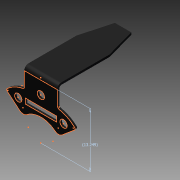
# Autodesk Inventor part: ASAP_Top_Fixture_Handle_New
Saved by Autodesk Inventor 2011 SP2 (Build 150309200, 309)
## iProperties
Created: 2011-11-18
Part Number: ASAP_Top_Fixture_Handle_New
Material: Default
Document SubType Name: Sheet Metal
Designer: sungwook
Density: 1 g/cm^3
Sheet Metal Rule: Default_mm
Flat Pattern Width: 1.65997 cm
Flat Pattern Length: 2.93845 cm
Flat Pattern Area: 4.87773 cm^2
Sheet Metal Width: 16.600 mm
Sheet Metal Length: 29.385 mm
Sheet Metal Area: 487.773 mm^2
Author: sungwook
Autodesk Inventor part; units mm, degrees
ref_plane "YZ Plane" through (0, 0, 0) normal (1, 0, 0) x (0, 1, 0)
ref_plane "XZ Plane" through (0, 0, 0) normal (0, 1, 0) x (-1, 0, 0)
ref_plane "XY Plane" through (0, 0, 0) normal (0, 0, 1) x (1, 0, 0)
sketch "Sketch1" plane through (0, 0, 0) normal (0, 0, 1) x (1, 0, 0)
  line L0 (-4, 10) -> (4, 10)
  line L1 (4, 10) -> (4, -10)
  line L2 (4, -10) -> (-4, -10)
  line L3 (-4, -10) -> (-4, 10)
  line L4 (-2, 10) -> (-4, 2.68)
  line L5 (0, -14) -> (0, 14)
  line L6 (2, 10) -> (4, 2.68)
  point P0 (0, 0)
  point P1 (0, 10)
  point P2 (-4, 0)
  dimension "d0" = 8
  dimension "d1" = 20
  dimension "d2" = 7.32
  dimension "d3" = 2
  dimension "d4" = 7.32
  dimension "d5" = 4
  measures "d0" distance between parallel lines of L1 L3
  measures "d1" distance between parallel lines of L2 L0
  measures "d2" vertical distance of L4.end L4.start
  measures "d3" distance of point (0, 10) L4.start
  measures "d4" vertical distance of L6.end L6.start
  measures "d5" distance of L6.start L4.start
extrude "Plate1" add sketch "Sketch1" along normal blind 0.508 contours L0 L5 L2 L3 L4 | L0 L6 L1 L2 L5
sketch "Sketch2" plane through (-4, -9.492, 0.508) normal (0, -1, 0) x (1, 0, 0)
  line L0 (8, 0) -> (0, 0)
  line L1 (0, 0) -> (0, -5)
  line L2 (0, -5) -> (8, -5)
  line L3 (8, -5) -> (8, 0)
  constraints: 4 end point, 4 other
edge flange "Flange1" height 5 angle 90 thickness 0.508 bend radius 0.508 thickness toward (0, -1, 0) relief straight relief width 0.508 relief depth 0.254 edges at (0, -10, 0) wall of the first edge with corners at (4, -9.492, 0.508) (-4, -9.492, 0.508) (-4, -9.492, -4.492) (4, -9.492, -4.492)
bend "Bend1"
corner "Corner1"
sketch "Block1" plane through (0, 0, 0) normal (0, 0, 1) x (1, 0, 0)
  line L0 (7.81, 3.3711) -> (7.81, 2.1011)
  circle A0 centre (12.3485, 0.5711) radius 0.5969
  arc A1 (12.9709, 2.3131) -> (7.0007, 5.198) centre (7.0007, -2.422) ccw
  arc A2 (14.6474, -0.5905) -> (12.9709, 2.3131) centre (4, -4.802) ccw
  circle A3 centre (10.0622, -0.7489) radius 0.8509
  line L1 (7.0007, 5.198) -> (0.9993, 5.198)
  arc A4 (14.1606, -7.2033) -> (14.6474, -0.5905) centre (7.5615, -3.3933) ccw
  line L2 (0.19, 2.1011) -> (0.19, 3.3711)
  line L3 (0.19, 3.3711) -> (7.81, 3.3711)
  line L4 (7.81, 2.1011) -> (0.19, 2.1011)
  arc A5 (7.9034, -8.1237) -> (9.3073, -5.692) centre (9.0593, -7.1699) ccw
  line L5 (11.1599, -12.4007) -> (14.1606, -7.2033)
  arc A6 (9.3073, -5.692) -> (7.9034, -8.1237) centre (4, -4.2489) ccw
  arc A7 (5.6764, -16.1286) -> (11.1599, -12.4007) centre (4.5608, -8.5907) ccw
  circle A8 centre (4, -11.2489) radius 0.8509
  circle A9 centre (4, -13.8889) radius 0.5969
  arc A10 (2.3236, -16.1286) -> (5.6764, -16.1286) centre (4, -4.802) ccw
  line L6 (-6.1606, -7.2033) -> (-3.1599, -12.4007)
  arc A11 (-3.1599, -12.4007) -> (2.3236, -16.1286) centre (3.4392, -8.5907) ccw
  arc A12 (0.9993, 5.198) -> (-4.9709, 2.3131) centre (0.9993, -2.422) ccw
  circle A13 centre (-2.0622, -0.7489) radius 0.8509
  arc A14 (-6.6474, -0.5905) -> (-6.1606, -7.2033) centre (0.4385, -3.3933) ccw
  arc A15 (-4.9709, 2.3131) -> (-6.6474, -0.5905) centre (4, -4.802) ccw
  circle A16 centre (-4.3485, 0.5711) radius 0.5969
  line L7 (4, -4.802) -> (4, 5.198)
  point P0 (4.4036, -3.4113)
sketch "Sketch13" plane through (-4, -10, -4.492) normal (0, -1, 0) x (1, 0, 0)
  line L0 (8, 3.984) -> (0, 3.984) projected
  line L1 (4, -27.1268) -> (4, 10.3545) projected
  circle A0 centre (4, -9.2649) radius 11.5
  line L2 (7.81, -1.6449) -> (7.81, -2.9149)
  circle A1 centre (12.3485, -4.4449) radius 0.5969
  arc A2 (12.9709, -2.7029) -> (7.0007, 0.182) centre (7.0007, -7.438) ccw
  arc A3 (14.6474, -5.6065) -> (12.9709, -2.7029) centre (4, -9.818) ccw
  circle A4 centre (10.0622, -5.7649) radius 0.8509
  line L3 (7.0007, 0.182) -> (0.9993, 0.182)
  arc A5 (14.1606, -12.2193) -> (14.6474, -5.6065) centre (7.5615, -8.4093) ccw
  line L4 (0.19, -2.9149) -> (0.19, -1.6449)
  line L5 (0.19, -1.6449) -> (7.81, -1.6449)
  line L6 (7.81, -2.9149) -> (0.19, -2.9149)
  arc A6 (7.9034, -13.1397) -> (9.3073, -10.708) centre (9.0593, -12.1859) ccw
  line L7 (11.1599, -17.4167) -> (14.1606, -12.2193)
  arc A7 (9.3073, -10.708) -> (7.9034, -13.1397) centre (4, -9.2649) ccw
  arc A8 (5.6764, -21.1446) -> (11.1599, -17.4167) centre (4.5608, -13.6067) ccw
  circle A9 centre (4, -16.2649) radius 0.8509
  circle A10 centre (4, -18.9049) radius 0.5969
  arc A11 (2.3236, -21.1446) -> (5.6764, -21.1446) centre (4, -9.818) ccw
  line L8 (-6.1606, -12.2193) -> (-3.1599, -17.4167)
  arc A12 (-3.1599, -17.4167) -> (2.3236, -21.1446) centre (3.4392, -13.6067) ccw
  arc A13 (0.9993, 0.182) -> (-4.9709, -2.7029) centre (0.9993, -7.438) ccw
  circle A14 centre (-2.0622, -5.7649) radius 0.8509
  arc A15 (-6.6474, -5.6065) -> (-6.1606, -12.2193) centre (0.4385, -8.4093) ccw
  arc A16 (-4.9709, -2.7029) -> (-6.6474, -5.6065) centre (4, -9.818) ccw
  circle A17 centre (-4.3485, -4.4449) radius 0.5969
  line L9 (4, -9.818) -> (4, 0.182)
  point P0 (4, 4.492)
  point P1 (4, 3.984)
  dimension "d79" = 3.802
  dimension "d83" = 13.249
  dimension "d110" = 23
  constraints: 1 centre point, 1 midpoint, 1 point on line, 1 other
  measures "d110" diameter of A0
sketch "Sketch15" plane through (-4, -10, -4.492) normal (0, -1, 0) x (1, 0, 0)
  line L0 (0, 0) -> (0, 3.984)
  arc A0 (9.3073, -10.708) -> (7.9034, -13.1397) centre (4, -9.2649) ccw
  arc A1 (0.9993, 0.182) -> (-4.9709, -2.7029) centre (0.9993, -7.438) ccw
  circle A2 centre (-4.3485, -4.4449) radius 0.5969
  circle A3 centre (-2.0622, -5.7649) radius 0.8509
  line L1 (4, -21.0244) -> (4, 9.3374)
  arc A4 (-4.125, -1.8061) -> (-4.165, -2.4137) centre (-3.9224, -2.1246) ccw
  arc A5 (-0.4226, 0.0482) -> (0, 0.5585) centre (-0.5195, 0.5585) ccw
  arc A6 (-1.1371, -4.9544) -> (0.5601, -4.9734) centre (-0.2769, -3.9292) ccw
  arc A7 (-0.4226, 0.0482) -> (-4.125, -1.8061) centre (1.0102, -7.4359) ccw
  line L2 (0, 0.5585) -> (4, 0.5585)
  arc A8 (4, -3.7649) -> (0.5601, -4.9734) centre (4, -9.2649) ccw
  line L3 (-1.1371, -4.9544) -> (-4.165, -2.4137)
  arc A9 (12.165, -2.4137) -> (12.125, -1.8061) centre (11.9224, -2.1246) ccw
  arc A10 (8, 0.5585) -> (8.4226, 0.0482) centre (8.5195, 0.5585) ccw
  arc A11 (7.4399, -4.9734) -> (9.1371, -4.9544) centre (8.2769, -3.9292) ccw
  arc A12 (12.125, -1.8061) -> (8.4226, 0.0482) centre (6.9898, -7.4359) ccw
  line L4 (8, 0.5585) -> (4, 0.5585)
  arc A13 (7.4399, -4.9734) -> (4, -3.7649) centre (4, -9.2649) ccw
  line L5 (9.1371, -4.9544) -> (12.165, -2.4137)
  line L6 (4, -9.2649) -> (-6.1438, -0.7533)
  point P0 (4, 4.492)
  dimension "d112" = 50
  measures "d112" angle of L1 L6
sheet face with bend "Face5" sketch "Sketch15" thickness 0.508 toward (0, 1, 0) bend radius 0.508 relief straight relief width 0.508 relief depth 0.254 contours A1 A5 L0 | L0 L2 L1 A0 A6 L3 A4 A7 A1 | A7 A4 A1 | L4 A10 A12 A9 L5 A11 A0 L1
bend "Bend6"
extrude "Cut2" cut sketch "Sketch13" against normal blind 0.508 contours L5 L2 L6 L1 | L1 L6 L4 L5
sketch "Sketch16" plane through (-4, -10, -0.508) normal (0, -1, 0) x (1, 0, 0)
  line L0 (4, -16.1019) -> (4, 3.869) projected
  point P0 (0.19, -6.8989)
  point P1 (4, 0.508)
  point P2 (-1.5, -6.3989)
  dimension "d92" = 5.5
  dimension "d94" = 0.5
  measures "d92" distance from line of L0 point (-1.5, -6.399)
  measures "d94" vertical distance of point (-1.5, -6.399) point (0.19, -6.899)
hole "Hole3" at (-5.5, -10, -6.9069) direction (0, 1, 0) diameter 1.778 end through all clearance for "Flat Head Machine Screw (82)" size "#0" standard "Ansi Unified Screw Threads"
mirror "Mirror2" about plane through (0, 0, 0) normal (1, 0, 0) of "Hole3"
sketch "Sketch17" plane through (-4, -10, -0.508) normal (0, -1, 0) x (1, 0, 0)
  line L0 (0.19, -5.6289) -> (7.81, -5.6289) projected
  point P0 (4, 0.508)
  point P1 (4, -3.1289)
  dimension "d102" = 2.5
  measures "d102" distance from line of point (4, -3.129) L0
hole "Hole4" at (0, -10, -3.6369) direction (0, 1, 0) diameter 1.778 end through all clearance for "Flat Head Machine Screw (82)" size "#0" standard "Ansi Unified Screw Threads"
sketch "Sketch18" plane through (-4, -10, -0.508) normal (0, -1, 0) x (1, 0, 0)
  circle A0 centre (4, -3.1289) radius 0.889 projected
  circle A1 centre (9.5, -6.3989) radius 0.889 projected
  circle A2 centre (-1.5, -6.3989) radius 0.889 projected
  line L0 (7.81, -5.6289) -> (7.81, -6.8989) projected
  line L1 (7.81, -6.8989) -> (0.19, -6.8989) projected
  line L2 (0.19, -6.8989) -> (0.19, -5.6289) projected
  line L3 (0.19, -5.6289) -> (7.81, -5.6289) projected
  line L4 (8, 0) -> (8, -3.4255) projected
  line L5 (8, 0) -> (0, 0) projected
  line L6 (0, -3.4255) -> (0, 0) projected
  arc A3 (-0.4226, -3.9358) -> (0, -3.4255) centre (-0.5195, -3.4255) ccw projected
  arc A4 (-0.4226, -3.9358) -> (-4.125, -5.7901) centre (1.0102, -11.4199) ccw projected
  arc A5 (-4.125, -5.7901) -> (-4.165, -6.3977) centre (-3.9224, -6.1086) ccw projected
  line L7 (-4.165, -6.3977) -> (-1.1371, -8.9384) projected
  arc A6 (-1.1371, -8.9384) -> (0.5601, -8.9574) centre (-0.2769, -7.9132) ccw projected
  arc A7 (7.4399, -8.9574) -> (0.5601, -8.9574) centre (4, -13.2489) ccw projected
  arc A8 (7.4399, -8.9574) -> (9.1371, -8.9384) centre (8.2769, -7.9132) ccw projected
  line L8 (9.1371, -8.9384) -> (12.165, -6.3977) projected
  arc A9 (12.165, -6.3977) -> (12.125, -5.7901) centre (11.9224, -6.1086) ccw projected
  arc A10 (12.125, -5.7901) -> (8.4226, -3.9358) centre (6.9898, -11.4199) ccw projected
  arc A11 (8, -3.4255) -> (8.4226, -3.9358) centre (8.5195, -3.4255) ccw projected
  point P0 (4, 0.508)
sketch "Sketch19" plane through (-4, -10, -0.508) normal (0, -1, 0) x (1, 0, 0)
  circle A0 centre (4, -3.1289) radius 0.889 projected
  circle A1 centre (9.5, -6.3989) radius 0.889 projected
  circle A2 centre (-1.5, -6.3989) radius 0.889 projected
  line L0 (7.81, -5.6289) -> (7.81, -6.8989) projected
  line L1 (7.81, -6.8989) -> (0.19, -6.8989) projected
  line L2 (0.19, -6.8989) -> (0.19, -5.6289) projected
  line L3 (0.19, -5.6289) -> (7.81, -5.6289) projected
  line L4 (8, 0) -> (8, -3.4255) projected
  line L5 (8, 0) -> (0, 0) projected
  line L6 (0, -3.4255) -> (0, 0) projected
  arc A3 (-0.4226, -3.9358) -> (0, -3.4255) centre (-0.5195, -3.4255) ccw projected
  arc A4 (-0.4226, -3.9358) -> (-4.125, -5.7901) centre (1.0102, -11.4199) ccw projected
  arc A5 (-4.125, -5.7901) -> (-4.165, -6.3977) centre (-3.9224, -6.1086) ccw projected
  line L7 (-4.165, -6.3977) -> (-1.1371, -8.9384) projected
  arc A6 (-1.1371, -8.9384) -> (0.5601, -8.9574) centre (-0.2769, -7.9132) ccw projected
  arc A7 (7.4399, -8.9574) -> (0.5601, -8.9574) centre (4, -13.2489) ccw projected
  arc A8 (7.4399, -8.9574) -> (9.1371, -8.9384) centre (8.2769, -7.9132) ccw projected
  line L8 (9.1371, -8.9384) -> (12.165, -6.3977) projected
  arc A9 (12.165, -6.3977) -> (12.125, -5.7901) centre (11.9224, -6.1086) ccw projected
  arc A10 (12.125, -5.7901) -> (8.4226, -3.9358) centre (6.9898, -11.4199) ccw projected
  arc A11 (8, -3.4255) -> (8.4226, -3.9358) centre (8.5195, -3.4255) ccw projected
  point P0 (4, 0.508)
  dimension "d113" = 13.249
  measures "d113" distance from line of A7.centre L5
equation "\"d110\" = baseOD"
equation "\"d90\" = Thickness"
equation "\"d100\" = Thickness"
equation "\"d108\" = Thickness"
equation "\"d7\" = BendReliefWidth"
equation "\"d8\" = BendReliefDepth"
equation "\"d9\" = MinimumRemnant"
equation "\"d10\" = BendRadius"
equation "\"d13\" = BendRadius"
equation "\"d14\" = CornerReliefSize"
equation "\"d15\" = GapSize"
equation "\"d16\" = JacobiRadiusSize"
equation "\"d85\" = BendRadius"
equation "\"d86\" = BendReliefWidth"
equation "\"d88\" = MinimumRemnant"
equation "\"d87\" = BendReliefDepth"
equation "\"d89\" = BendRadius"
equation "\"BendRadius\" = Thickness"
equation "\"BendReliefWidth\" = Thickness"
equation "\"BendReliefDepth\" = 0.5 * Thickness"
equation "\"CornerReliefSize\" = 4 * Thickness"
equation "\"MinimumRemnant\" = 2 * Thickness"
equation "\"TransitionRadius\" = BendRadius"
equation "\"JacobiRadiusSize\" = BendRadius"
equation "\"GapSize\" = Thickness"
equation "\"d6\" = BendRadius"
equation "\"baseOD\" = 23"
equation "\"baseInitD\" = 4"
equation "\"baseTh0\" = 48.463041deg"
equation "\"baseTh1\" = 23.073918deg"
equation "\"topD\" = 14"
equation "\"topInitD\" = 4"
equation "\"topTh0\" = 16.60155deg"
equation "\"topTh1\" = 86.796901deg"
equation "\"dFlexure\" = 0.38"
equation "\"lFlexure\" = 6.7"
equation "\"lFlexureOffset\" = 3.7"
equation "\"dMotor\" = 1.44"
equation "\"lMotor\" = 22.35"
equation "\"topH\" = 21.66629"
equation "\"springBaseD\" = 8"
equation "\"springTopD\" = 8"
equation "\"springInitL\" = 12.7"
equation "\"springLset\" = 3.5"
equation "\"springDeform\" = 18.16629"
equation "\"springL\" = 30.86629"
equation "\"springLO\" = 33.86629"
equation "\"springUnderCut\" = 9.2"
equation "\"dM1X\" = 6.73587"
equation "\"dM1Y\" = 2.34012"
equation "\"dM2X\" = -1.34133"
equation "\"dM2Y\" = 7.00349"
equation "\"dM1Xt\" = 6.59227"
equation "\"dM1Yt\" = -0.43704"
equation "\"dM2Xt\" = -3.67462"
equation "\"dM2Yt\" = 5.49055"
equation "\"GuideRod\" = 2"
equation "\"GuideTubingOD\" = 4"
equation "\"GuideTubingID\" = 2"
equation "\"CSpringOD\" = 5.537"
equation "\"CSpringCD\" = 0.254"
equation "\"CSpringID\" = 5.029"
equation "\"Thickness\" = 0.508"
body "Solid1"
